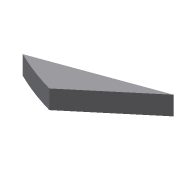
# Autodesk Inventor part: Vane_blade
Saved by Autodesk Inventor 2022 (Build 260148000, 148)
## iProperties
Created: 2005-10-19
Part Number: Vane_blade
Document SubType Name: Modeling
Designer: landrews
Density: 1 g/cm^3
Material: Generic
Appearance: Default
Author: landrews
Autodesk Inventor part; units mm, degrees
ref_plane "YZ Plane" through (0, 0, 0) normal (1, 0, 0) x (0, 1, 0)
ref_plane "XZ Plane" through (0, 0, 0) normal (0, 1, 0) x (-1, 0, 0)
ref_plane "XY Plane" through (0, 0, 0) normal (0, 0, 1) x (1, 0, 0)
sketch "Sketch1" plane through (0, 0, 0) normal (0, 1, 0) x (-1, 0, 0)
  line L0 (-16.0222, 0) -> (58.748, 0) projected
  line L1 (0, -100.5662) -> (0, 62.7605) projected
  arc A0 (53.2252, 19.3751) -> (32.5174, 27.2854) centre (0, -88.9) ccw
  line L2 (0, 0) -> (32.5174, 27.2854)
  line L3 (0, 0) -> (53.2252, 19.3751)
  dimension "d5" = 50
  dimension "d6" = 69.997
  dimension "d7" = 56.642
  dimension "d8" = 42.4485
  constraints: 4 end point, 2 point on circle, 2 point on line, 1 centre point
  measures "d5" angle of L1 L2
  measures "d6" angle of L1 L3
  measures "d7" distance of L2.start L3.end
  measures "d8" distance of L2.start L2.end
extrude "Extrusion1" add sketch "Sketch1" along normal blind 9.017
body "Solid1"
